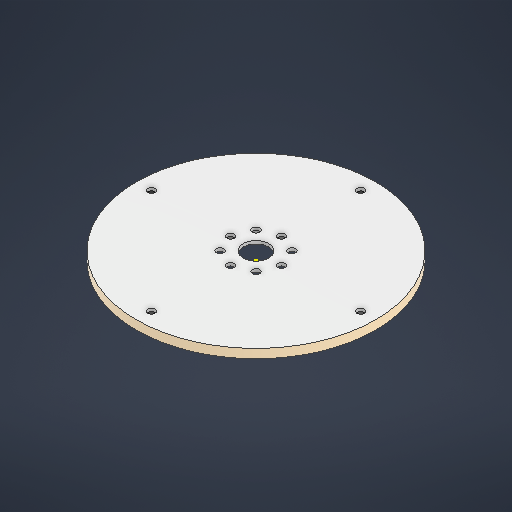
# Autodesk Inventor part: spool_test
Saved by Autodesk Inventor 2026.2 (Build 302298010, 298A)
## iProperties
Created: 2026-02-24
Part Number: spool_test
Material: ABS Plastic
Document SubType Name: Modeling
Designer: Luke
Density: 1.06 g/cm^3
Appearance: Smooth - White
Author: Luke
Autodesk Inventor part; units mm, degrees
ref_plane "YZ Plane" through (0, 0, 0) normal (1, 0, 0) x (0, 1, 0)
ref_plane "XZ Plane" through (0, 0, 0) normal (0, 1, 0) x (-1, 0, 0)
ref_plane "XY Plane" through (0, 0, 0) normal (0, 0, 1) x (1, 0, 0)
sketch "Sketch1" plane through (0, 0, 0) normal (0, 1, 0) x (-1, 0, 0)
  circle A0 centre (0, 0) radius 30
  circle A1 centre (0, 0) radius 45
  circle A2 centre (0, 0) radius 20
  dimension "d0" = 60
  dimension "d1" = 90
  dimension "d2" = 40
  constraints: 3 centre point, 3 coincident
  measures "d0" diameter of A0
  measures "d1" diameter of A1
  measures "d2" diameter of A2
extrude "Extrusion1" add sketch "Sketch1" along normal blind 20 draft -4 contours A0
sketch "Sketch2" plane through (0, 20, 0) normal (0, 1, 0) x (1, 0, 0)
  circle A0 centre (0, 0) radius 28.6015
  circle A1 centre (0, 0) radius 21.3985
  constraints: 2 centre point, 2 coincident
extrude "Extrusion2" add sketch "Sketch2" along normal blind 20 draft 4
sketch "Sketch3" plane through (0, 40, 0) normal (0, 1, 0) x (1, 0, 0)
  circle A0 centre (0, 0) radius 40
  dimension "d7" = 80
  constraints: 1 centre point, 1 coincident
  measures "d7" diameter of A0
extrude "Extrusion3" add sketch "Sketch3" along normal blind 10
sketch "Sketch4" plane through (0, 0, 0) normal (0, -1, 0) x (1, 0, 0)
  circle A0 centre (0, 0) radius 40
  dimension "d10" = 80
  constraints: 1 centre point, 1 coincident
  measures "d10" diameter of A0
extrude "Extrusion4" add sketch "Sketch4" along normal blind 10
sketch "Sketch5" plane through (0, -10, 0) normal (0, -1, 0) x (1, 0, 0)
  circle A0 centre (0, 0) radius 2.25
  circle A1 centre (0, 0) radius 4.25
  circle A2 centre (0, 0) radius 10.25
  dimension "d13" = 4.5
  dimension "d16" = 8.5
  dimension "d17" = 20.5
  constraints: 3 centre point, 3 coincident
  measures "d13" diameter of A0
  measures "d16" diameter of A1
  measures "d17" diameter of A2
extrude "Extrusion9" cut sketch "Sketch5" against normal blind 2 contours A2
extrude "Extrusion10" cut sketch "Sketch5" against normal blind 4 contours A0 | A1
sketch "Sketch6" plane through (0, -8, 0) normal (0, -1, 0) x (1, 0, 0)
  circle A0 centre (0, 8.5) radius 1.25
  circle A1 centre (0, 0) radius 8.5
  circle A2 centre (-6.0104, 6.0104) radius 1.25
  circle A3 centre (-8.5, 0) radius 1.25
  circle A4 centre (-6.0104, -6.0104) radius 1.25
  circle A5 centre (0, -8.5) radius 1.25
  circle A6 centre (6.0104, -6.0104) radius 1.25
  circle A7 centre (8.5, 0) radius 1.25
  circle A8 centre (6.0104, 6.0104) radius 1.25
  circle A9 centre (0, 0) radius 10.25 projected
  line L0 (0, 8.5) -> (0, 7.25) construction
  line L1 (0, -8.5) -> (0, -7.25) construction
  line L2 (0, 7.25) -> (0, 0) construction
  point P0 (5.0639, 6.8269)
  point P1 (6.8269, 5.0639)
  dimension "d34" = 2.5
  dimension "d30" = 360
  dimension "d36" = 14.5
  dimension "d37" = 1.25
  constraints: 7 centre point, 6 end point, 3 vertical, 2 point on circle, 2 vertical alignment, 1 coincident, 21 other
  measures "d36" distance of L1.end L0.end
  measures "d37" distance of L1.start L1.end
extrude "Extrusion11" cut sketch "Sketch6" against normal through all contours A0 A1 | A1 A0 | A2 A1 | A1 A2 | A8 A1 | A1 A8 | A3 A1 | A1 A3 | A7 A1 | A1 A7 | A4 A1 | A1 A4 | A6 A1 | A1 A6 | A5 A1 | A1 A5
sketch "Sketch7" plane through (0, -10, 0) normal (0, -1, 0) x (1, 0, 0)
  point P0 (0, 0)
sketch "Sketch8" plane through (0, 50, 0) normal (0, 1, 0) x (1, 0, 0)
  circle A0 centre (0, 0) radius 69.6174
  constraints: 1 centre point, 1 coincident
extrude "Extrusion12" cut sketch "Sketch8" against normal blind 57
sketch "Sketch12" plane through (0, -10, 0) normal (0, -1, 0) x (1, 0, 0)
  circle A0 centre (0, 0) radius 4.25 projected
  circle A1 centre (0, 0) radius 35 construction
  point P0 (0, 35)
  dimension "d57" = 70
  constraints: 1 coincident, 1 vertical alignment, 2 other
hole "Hole2" at (0, -10, 35) direction (0, 1, 0) diameter 2.5 depth 8 tip angle 118 counterbore diameter 5 counterbore depth 2
pattern_circular "Circular Pattern2" count 4 over 360 about axis through (0, 0, 0) along (0, -1, 0) of "Hole2"
sketch "Sketch9" plane through (0, -10, 0) normal (0, -1, 0) x (1, 0, 0)
  circle A0 centre (0, 0) radius 16.7725
  circle A1 centre (0, 0) radius 4.25 projected
  circle A2 centre (0, 0) radius 45.7596
  constraints: 2 centre point, 2 coincident
body "Solid1"
